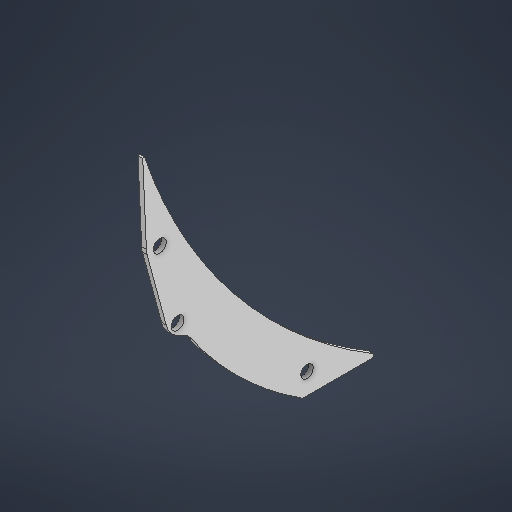
# Autodesk Inventor part: ramps
Saved by Autodesk Inventor 2025.2 (Build 292293000, 293)
## iProperties
Created: 2025-04-06
Part Number: ramps
Material: Generic
Document SubType Name: Modeling
Designer: roejo
Density: 1 g/cm^3
Appearance: Default
Author: roejo
Autodesk Inventor part; units mm, degrees
ref_plane "YZ Plane" through (0, 0, 0) normal (1, 0, 0) x (0, 1, 0)
ref_plane "XZ Plane" through (0, 0, 0) normal (0, 1, 0) x (-1, 0, 0)
ref_plane "XY Plane" through (0, 0, 0) normal (0, 0, 1) x (1, 0, 0)
sketch "Sketch1" plane through (0, 0, 0) normal (1, 0, 0) x (0, 1, 0)
  arc A0 (-5.9812, 90.4765) -> (-7.6488, 90.2536) centre (-5.9812, 84.1265) ccw
  line L0 (-31.2813, 83.8216) -> (-7.6488, 90.2536)
  arc A1 (-31.2813, 83.8216) -> (-36.6872, 78.9462) centre (-29.7456, 76.684) ccw
  arc A2 (-39.1231, 75.684) -> (-36.6872, 78.9462) centre (-42.7247, 80.9138) ccw
  circle A3 centre (-32.5683, 80.0194) radius 2.1844
  line L1 (-68.3342, 42.995) -> (-68.3342, 36.645)
  circle A4 centre (-68.3342, 36.645) radius 2.0955
  line L2 (-75.4217, 14.8355) -> (-75.4217, 38.0637)
  arc A5 (-39.1231, 75.684) -> (-75.4217, 38.0637) centre (35.426, -32.5681) ccw
  arc A6 (-75.4217, 14.8355) -> (-74.2538, 14.4902) centre (-74.7867, 14.8355) ccw
  line L3 (-5.9812, 90.4765) -> (20.9089, 91.6876)
  arc A7 (21.0249, 91.0696) -> (-74.2538, 14.4902) centre (77.9842, -77.3598) ccw
  circle A8 centre (-7.2163, 86.0118) radius 2.1844
  arc A9 (21.0249, 91.0696) -> (20.9089, 91.6876) centre (20.9232, 91.3704) ccw
  point P0 (0, 0)
  point P1 (-4.9764, 91.8669)
  point P2 (-75.4217, 12.6637)
  point P3 (23.2041, 91.791)
  point P4 (-74.2538, 14.4902)
  dimension "d1" = 4.191
  dimension "d4" = 25.4
  dimension "d5" = 0.635
  dimension "d9" = 177.8
  dimension "d10" = 4.3688
  dimension "d11" = 0.3175
  constraints: 15 point on circle, 10 centre point, 8 end point, 4 tangent, 2 point on line, 1 coincident, 1 vertical
  measures "d1" diameter of A4
  measures "d4" distance of point (-75.422, 12.664) L2.end
  measures "d5" radius of A6
  measures "d9" radius of A7
  measures "d10" diameter of A8
  measures "d11" radius of A9
extrude "Extrusion1" add sketch "Sketch1" along normal blind 1.5875
body "Solid1"
